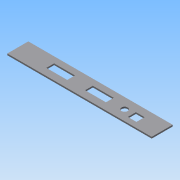
# Autodesk Inventor part: panel 2
Saved by Autodesk Inventor 2013 (Build 170138000, 138)
## iProperties
Created: 2014-07-23
Part Number: panel 2
Material: Generic
Document SubType Name: Sheet Metal
Designer: User
Density: 1 g/cm^3
Sheet Metal Rule: Default_mm
Author: User
Autodesk Inventor part; units mm, degrees
ref_plane "YZ Plane" through (0, 0, 0) normal (1, 0, 0) x (0, 1, 0)
ref_plane "XZ Plane" through (0, 0, 0) normal (0, 1, 0) x (-1, 0, 0)
ref_plane "XY Plane" through (0, 0, 0) normal (0, 0, 1) x (1, 0, 0)
sketch "Sketch1" plane through (0, 0, 0) normal (0, 0, 1) x (1, 0, 0)
  circle A0 centre (76.6657, 1.1203) radius 3
  line L0 (88.1657, -4.2797) -> (97.1657, -4.2797)
  line L1 (97.1657, -4.2797) -> (97.1657, 4.1203)
  line L2 (97.1657, 4.1203) -> (88.1657, 4.1203)
  line L3 (124.4657, -12.1297) -> (124.4657, 14.6703)
  line L4 (88.1657, 4.1203) -> (88.1657, -4.2797)
  line L5 (56.0657, -2.0797) -> (56.0657, 5.8203)
  line L6 (33.6679, 7.1494) -> (33.6679, -2.7506)
  line L7 (32.8657, 14.6703) -> (32.8657, -12.1297)
  line L8 (31.4657, -2.0797) -> (56.0657, -2.0797)
  line L9 (56.0657, 5.8203) -> (31.4657, 5.8203)
  line L10 (124.4657, 14.6703) -> (-59.7343, 14.6703)
  line L11 (-59.7343, -5.3797) -> (124.4657, -5.3797)
  line L12 (-59.7343, -12.1297) -> (124.4657, -12.1297)
  line L13 (31.4657, 5.8203) -> (31.4657, -2.0797)
  line L14 (-59.7343, 14.6703) -> (-59.7343, -12.1297)
  line L15 (6.6657, -2.0797) -> (6.6657, 5.8203)
  line L16 (-17.9343, -2.0797) -> (6.6657, -2.0797)
  line L17 (-17.9343, 5.8203) -> (-17.9343, -2.0797)
  line L18 (6.6657, 5.8203) -> (-17.9343, 5.8203)
  line L19 (7.6657, 6.8203) -> (7.6657, -3.0797)
  line L20 (7.6657, -3.0797) -> (-18.9343, -3.0797)
  line L21 (-18.9343, -3.0797) -> (-18.9343, 6.8203)
  line L22 (-18.9343, 6.8203) -> (7.6657, 6.8203)
  line L23 (57.0657, 6.8203) -> (57.0657, -3.0797)
  line L24 (57.0657, -3.0797) -> (30.4657, -3.0797)
  line L25 (30.4657, -3.0797) -> (30.4657, 6.8203)
  line L26 (30.4657, 6.8203) -> (57.0657, 6.8203)
  circle A1 centre (76.6657, 1.1203) radius 4
  line L27 (98.1657, 5.1203) -> (98.1657, -5.2797)
  line L28 (98.1657, -5.2797) -> (87.1657, -5.2797)
  line L29 (87.1657, -5.2797) -> (87.1657, 5.1203)
  line L30 (87.1657, 5.1203) -> (98.1657, 5.1203)
  point P0 (0, 0)
  point P1 (0, 0)
  dimension "d1" = 6.75
  dimension "d2" = 7.9
  dimension "d3" = 24.6
  dimension "d4" = 3.3
  dimension "d5" = 3.3
  dimension "d6" = 24.6
  dimension "d7" = 7.9
  dimension "d8" = 24.8
  dimension "d10" = 6
  dimension "d11" = 6.5
  dimension "d12" = 20.6
  dimension "d13" = 9
  dimension "d14" = 1.1
  dimension "d15" = 8.4
  dimension "d17" = 1
  dimension "d18" = 1
  dimension "d19" = 1
  dimension "d20" = 1
  dimension "d27" = 11.5
  dimension "d30" = 26.8
  dimension "d32" = 41.8
  dimension "d33" = 184.2
  constraints: 62 end point, 12 parallel, 8 perpendicular, 5 point on line, 3 horizontal, 2 centre point, 9 other
  measures "d1" distance between parallel lines of L12 L11
  measures "d2" distance between parallel lines of L18 L16
  measures "d3" distance of L18.start L17.start
  measures "d4" distance between parallel lines of L11 L16
  measures "d5" distance between parallel lines of L11 L8
  measures "d6" distance of L5.end L9.end
  measures "d7" distance between parallel lines of L9 L8
  measures "d8" distance between parallel lines of L13 L15
  measures "d10" diameter of A0
  measures "d11" distance from line of L11 A0.centre
  measures "d12" distance from line of A0.centre L5
  measures "d13" distance of L1.end L4.start
  measures "d14" distance between parallel lines of L11 L0
  measures "d15" distance of L0.end L1.end
  measures "d17" distance between parallel lines of L19 L15
  measures "d18" distance between parallel lines of L23 L5
  measures "d19" radial gap between concentric circles of A1 A0
  measures "d20" distance between parallel lines of L27 L1
  measures "d27" distance from line of L4 A0.centre
  measures "d30" distance of L12.end L10.start
  measures "d32" distance between parallel lines of L17 L14
  measures "d33" distance of L12.start L12.end
extrude "Extrusion1" add sketch "Sketch1" along normal blind 1.9 contours L12 L7 L11 L3 | L11 L7 L24 L23 L26 L10 L3 | L12 L14 L11 L7 | L11 L14 L10 L7 L26 L25 L24
equation "\"BendRadius\" = Thickness"
equation "\"BendReliefWidth\" = Thickness"
equation "\"BendReliefDepth\" = 0.5 * Thickness"
equation "\"CornerReliefSize\" = 4 * Thickness"
equation "\"MinimumRemnant\" = 2 * Thickness"
equation "\"TransitionRadius\" = BendRadius"
equation "\"JacobiRadiusSize\" = BendRadius"
equation "\"GapSize\" = Thickness"
equation "\"Thickness\" = 0.5"
body "Solid1"
